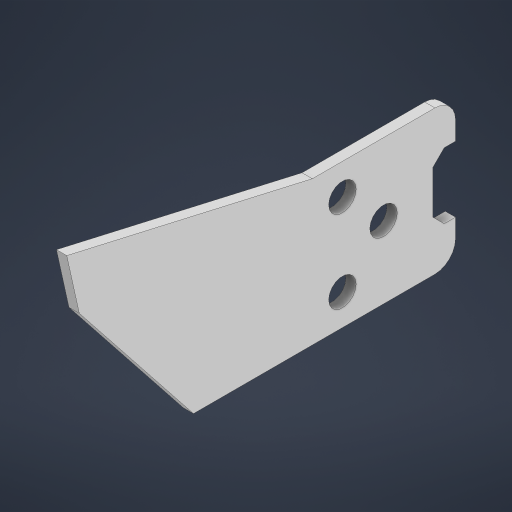
# Autodesk Inventor part: sled
Saved by Autodesk Inventor 2024 (Build 280153000, 153)
## iProperties
Created: 2023-08-09
Part Number: sled
Material: Generic
Document SubType Name: Modeling
Designer: macbook
Density: 1 g/cm^3
Appearance: Default
Author: macbook
Autodesk Inventor part; units mm, degrees
ref_plane "YZ Plane" through (0, 0, 0) normal (1, 0, 0) x (0, 1, 0)
ref_plane "XZ Plane" through (0, 0, 0) normal (0, 1, 0) x (-1, 0, 0)
ref_plane "XY Plane" through (0, 0, 0) normal (0, 0, 1) x (1, 0, 0)
sketch "Sketch1" plane through (0, 0, 0) normal (1, 0, 0) x (0, 1, 0)
  line L0 (22.225, -19.05) -> (22.225, -2.4283)
  arc A0 (0, -19.05) -> (3.175, -22.225) centre (3.175, -19.05) ccw
  arc A1 (19.05, -22.225) -> (22.225, -19.05) centre (19.05, -19.05) ccw
  line L1 (22.225, -2.4283) -> (22.225, -0.1256)
  line L2 (0, 9.3994) -> (0, -19.05)
  line L3 (0, 9.3994) -> (0, 18.2179)
  line L4 (0, 18.2179) -> (22.225, 35.8469)
  line L5 (22.225, 35.8469) -> (30.8968, 37.7761)
  line L6 (30.8968, 37.7761) -> (22.225, -0.1256)
  line L7 (11.1125, -18.7325) -> (14.4463, -18.7325)
  line L8 (16.1925, -22.225) -> (19.05, -22.225)
  line L9 (6.0325, -22.225) -> (3.175, -22.225)
  line L10 (16.1925, -20.4788) -> (14.4463, -18.7325)
  line L11 (16.1925, -20.4788) -> (16.1925, -22.225)
  line L12 (14.4463, -18.7325) -> (7.7787, -18.7325)
  line L13 (6.0325, -20.4788) -> (7.7787, -18.7325)
  line L14 (6.0325, -20.4788) -> (6.0325, -22.225)
  line L15 (11.1125, -0.1256) -> (11.1125, -4.8881)
  line L16 (11.1125, -4.8881) -> (11.1125, -17.5881)
  line L17 (11.1125, -17.5881) -> (17.4625, -17.5881)
  line L18 (17.4625, -17.5881) -> (4.7625, -17.5881)
  line L19 (17.4625, -18.6041) -> (17.4625, -15.5561)
  line L20 (4.7625, -18.6041) -> (4.7625, -15.5561)
  point P0 (0, -22.225)
  point P1 (22.225, -22.225)
  point P2 (22.225, 31.6244)
  dimension "d1" = 22.225
  dimension "d6" = 3.175
  dimension "d27" = 31.75
  dimension "d32" = 4.7625
  dimension "d40" = 3.048
  dimension "d41" = 3.048
  constraints: 42 end point, 5 point on line, 4 perpendicular, 4 point on circle, 4 vertical, 2 centre point, 1 equal radius, 1 horizontal, 1 tangent
  measures "d1" distance of point (0, -22.225) point (22.225, -22.225)
  measures "d6" radius of A0
  measures "d27" distance of L1.end point (22.225, 31.624)
  measures "d32" distance of L15.start L15.end
  measures "d40" distance of L19.start L19.end
  measures "d41" distance of L20.start L20.end
extrude "Extrusion1" add sketch "Sketch1" along normal blind 1.5875
sketch "Sketch2" plane through (1.5875, 0, 0) normal (1, 0, 0) x (0, 0, -1)
  line L0 (22.225, 3.175) -> (22.225, 19.05) projected
  line L1 (0, 11.1125) -> (4.7625, 11.1125)
  line L2 (4.7625, 11.1125) -> (17.4625, 11.1125)
  line L3 (17.4625, 11.1125) -> (22.225, 11.1125)
  line L4 (4.7625, 11.1125) -> (4.7625, 17.4625)
  line L5 (17.4625, 17.4625) -> (17.4625, 4.7625)
  line L6 (4.7625, 4.7625) -> (4.7625, 11.1125)
  point P0 (0, 0)
  point P1 (11.1125, 11.1125)
  dimension "d13" = 4.7625
  dimension "d14" = 12.7
  dimension "d15" = 6.35
  dimension "d16" = 12.7
  constraints: 12 end point, 2 coincident, 2 midpoint, 2 vertical, 1 horizontal, 1 perpendicular
  measures "d13" distance of L1.start L1.end
  measures "d14" distance of L1.end L2.end
  measures "d15" distance of L1.end L4.end
  measures "d16" distance of L5.start L5.end
hole "Hole1" at (1.5875, 17.4625, -4.7625) at (1.5875, 4.7625, -4.7625) at (1.5875, 11.1125, -11.1125) direction (-1, 0, 0) diameter 4.2418 end through all
body "Solid1"
